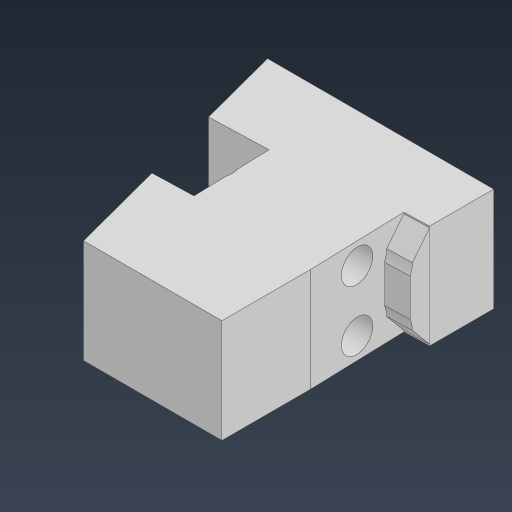
# Autodesk Inventor part: lunas_hold
Saved by Autodesk Inventor 2023 (Build 270158000, 158)
## iProperties
Created: 2026-01-11
Part Number: lunas_hold
Material: Generic
Document SubType Name: Modeling
Designer: szymo
Density: 1 g/cm^3
Appearance: Default
Author: szymo
Autodesk Inventor part; units mm, degrees
ref_plane "YZ Plane" through (0, 0, 0) normal (1, 0, 0) x (0, 1, 0)
ref_plane "XZ Plane" through (0, 0, 0) normal (0, 1, 0) x (-1, 0, 0)
ref_plane "XY Plane" through (0, 0, 0) normal (0, 0, 1) x (1, 0, 0)
ref_plane "Work Plane3" through (-37.2395, -29.2125, 19.3676) normal (0, -1, 0) x (0.9995066, 0, -0.0314108)
sketch "Sketch1" plane through (-37.2395, -29.2125, 19.3676) normal (0, -1, 0) x (0.9995066, 0, -0.0314108)
  line L0 (12, -4) -> (1, -4) construction
  line L1 (1, -4) -> (1, -14) construction
  line L2 (1, -14) -> (12, -14) construction
  line L3 (12, -14) -> (12, -13.8653) construction
  line L4 (10, -13.8653) -> (12, -13.8653) construction
  line L5 (10, -6.1347) -> (10, -13.8653) construction
  line L6 (10, -6.1347) -> (12, -6.1347) construction
  line L7 (12, -6.1347) -> (12, -4) construction
  line L8 (-5.9357, -19.5637) -> (1.1024, 11.0154) projected
  line L9 (1.1024, 11.0154) -> (32.2008, 11.9927) projected
  line L10 (33.1539, -18.3352) -> (32.2008, 11.9927) projected
  line L11 (33.1539, -18.3352) -> (-5.9357, -19.5637) projected
  line L12 (12.1612, -18.9949) -> (12, -13.8653)
  line L13 (12, -13.8653) -> (10, -13.8653)
  line L14 (10, -13.8653) -> (10, -6.1347)
  line L15 (10, -6.1347) -> (9.7777, 0.94)
  line L16 (-1.3163, -3.952) -> (-2.2908, -3.7277)
  line L17 (9.7777, 0.94) -> (-1.2966, 0.592)
  point P0 (37.8294, -18.1883)
  dimension "d0" = 20
  constraints: 12 end point, 2 perpendicular, 2 point on line, 1 collinear, 1 parallel, 3 other
  measures "d0" distance between parallel lines of L11 L17
extrude "Extrusion1" add sketch "Sketch1" along normal blind 8.3 contours L8 L17 L15 L14 L13 L12 L11
sketch "Sketch2" plane through (-27.4371, -37.5125, 12.9217) normal (0.9995066, 0, -0.0314108) x (-0.0314108, 0, -0.9995066)
  line L0 (7.7305, 8.3) -> (0, 8.3) projected
  line L1 (0, 8.3) -> (0, 0) projected
  line L2 (7.7305, 0) -> (0, 0) projected
  line L3 (7.7305, 8.3) -> (7.7305, 0) projected
  line L4 (-7.2847, -18.775) -> (-8.2847, -18.775) projected
  line L5 (-8.2847, -22.025) -> (-8.2847, -18.775) projected
  arc A0 (-8.2847, -22.025) -> (-7.7847, -22.525) centre (-7.7847, -22.025) ccw projected
  line L6 (-7.7847, -22.525) -> (-6.6313, -22.525) projected
  arc A1 (-6.1317, -23.0056) -> (-6.6313, -22.525) centre (-6.6313, -23.025) ccw projected
  arc A2 (-6.1317, -23.0056) -> (-2.1347, -26.85) centre (-2.1347, -22.85) ccw projected
  line L7 (0, -26.85) -> (-2.1347, -26.85) projected
  line L8 (1.6153, -28.775) -> (0, -26.85) projected
  arc A3 (1.6153, -28.775) -> (6.1153, -28.775) centre (3.8653, -28.775) ccw projected
  line L9 (7.7305, -26.85) -> (6.1153, -28.775) projected
  line L10 (7.8653, -26.85) -> (7.7305, -26.85) projected
  arc A4 (7.8653, -26.85) -> (12.8653, -21.85) centre (7.8653, -21.85) ccw projected
  line L11 (12.8653, -5.2) -> (12.8653, -21.85) projected
  arc A5 (12.8653, -5.2) -> (7.8653, -0.2) centre (7.8653, -5.2) ccw projected
  line L12 (7.7305, -0.2) -> (7.8653, -0.2) projected
  line L13 (6.1153, 1.725) -> (7.7305, -0.2) projected
  arc A6 (6.1153, 1.725) -> (1.6153, 1.725) centre (3.8653, 1.725) ccw projected
  line L14 (0, -0.2) -> (1.6153, 1.725) projected
  line L15 (-2.1347, -0.2) -> (0, -0.2) projected
  arc A7 (-2.1347, -0.2) -> (-6.1317, -4.0444) centre (-2.1347, -4.2) ccw projected
  arc A8 (-6.6313, -4.525) -> (-6.1317, -4.0444) centre (-6.6313, -4.025) ccw projected
  line L16 (-7.7847, -4.525) -> (-6.6313, -4.525) projected
  arc A9 (-7.7847, -4.525) -> (-8.2847, -5.025) centre (-7.7847, -5.025) ccw projected
  line L17 (-8.2847, -8.275) -> (-8.2847, -5.025) projected
  line L18 (-7.2847, -8.275) -> (-8.2847, -8.275) projected
  line L19 (-7.2847, -18.775) -> (-7.2847, -8.275) projected
  circle A10 centre (3.8653, -28.775) radius 1.1 projected
  circle A11 centre (3.8653, 1.725) radius 1.1 projected
  line L20 (-7.2847, 16.575) -> (-8.2847, 16.575) projected
  line L21 (-8.2847, 13.325) -> (-8.2847, 16.575) projected
  arc A12 (-8.2847, 13.325) -> (-7.7847, 12.825) centre (-7.7847, 13.325) ccw projected
  line L22 (-7.7847, 12.825) -> (-6.6313, 12.825) projected
  arc A13 (-6.1317, 12.3444) -> (-6.6313, 12.825) centre (-6.6313, 12.325) ccw projected
  arc A14 (-6.1317, 12.3444) -> (-2.1347, 8.5) centre (-2.1347, 12.5) ccw projected
  line L23 (0, 8.5) -> (-2.1347, 8.5) projected
  line L24 (1.6153, 6.575) -> (0, 8.5) projected
  arc A15 (1.6153, 6.575) -> (6.1153, 6.575) centre (3.8653, 6.575) ccw projected
  line L25 (7.7305, 8.5) -> (6.1153, 6.575) projected
  line L26 (7.8653, 8.5) -> (7.7305, 8.5) projected
  arc A16 (7.8653, 8.5) -> (12.8653, 13.5) centre (7.8653, 13.5) ccw projected
  line L27 (12.8653, 30.15) -> (12.8653, 13.5) projected
  arc A17 (12.8653, 30.15) -> (7.8653, 35.15) centre (7.8653, 30.15) ccw projected
  line L28 (7.7305, 35.15) -> (7.8653, 35.15) projected
  line L29 (6.1153, 37.075) -> (7.7305, 35.15) projected
  arc A18 (6.1153, 37.075) -> (1.6153, 37.075) centre (3.8653, 37.075) ccw projected
  line L30 (0, 35.15) -> (1.6153, 37.075) projected
  line L31 (-2.1347, 35.15) -> (0, 35.15) projected
  arc A19 (-2.1347, 35.15) -> (-6.1317, 31.3056) centre (-2.1347, 31.15) ccw projected
  arc A20 (-6.6313, 30.825) -> (-6.1317, 31.3056) centre (-6.6313, 31.325) ccw projected
  line L32 (-7.7847, 30.825) -> (-6.6313, 30.825) projected
  arc A21 (-7.7847, 30.825) -> (-8.2847, 30.325) centre (-7.7847, 30.325) ccw projected
  line L33 (-8.2847, 27.075) -> (-8.2847, 30.325) projected
  line L34 (-7.2847, 27.075) -> (-8.2847, 27.075) projected
  line L35 (-7.2847, 16.575) -> (-7.2847, 27.075) projected
  circle A22 centre (3.8653, 6.575) radius 1.1 projected
  circle A23 centre (3.8653, 37.075) radius 1.1 projected
  arc A24 (6.3141, 1.7991) -> (1.4164, 1.7991) centre (3.8653, 1.725) ccw
  line L36 (6.3141, 1.7991) -> (7.8238, 0)
  line L37 (7.8238, 0) -> (7.8653, 0)
  arc A25 (13.0653, -5.2) -> (7.8653, 0) centre (7.8653, -5.2) ccw
  line L38 (13.0653, -5.2) -> (13.0653, -21.85)
  arc A26 (7.8653, -27.05) -> (13.0653, -21.85) centre (7.8653, -21.85) ccw
  line L39 (7.8653, -27.05) -> (7.8238, -27.05)
  line L40 (7.8238, -27.05) -> (6.3141, -28.8491)
  arc A27 (1.4164, -28.8491) -> (6.3141, -28.8491) centre (3.8653, -28.775) ccw
  line L41 (1.4164, -28.8491) -> (-0.0933, -27.05)
  line L42 (-0.0933, -27.05) -> (-2.1347, -27.05)
  arc A28 (-6.3316, -23.0133) -> (-2.1347, -27.05) centre (-2.1347, -22.85) ccw
  arc A29 (-6.3316, -23.0133) -> (-6.6313, -22.725) centre (-6.6313, -23.025) ccw
  line L43 (-6.6313, -22.725) -> (-7.7847, -22.725)
  arc A30 (-8.4847, -22.025) -> (-7.7847, -22.725) centre (-7.7847, -22.025) ccw
  line L44 (-8.4847, -22.025) -> (-8.4847, -18.575)
  line L45 (-8.4847, -18.575) -> (-7.4847, -18.575)
  line L46 (-7.4847, -18.575) -> (-7.4847, -8.475)
  line L47 (-7.4847, -8.475) -> (-8.4847, -8.475)
  line L48 (-8.4847, -8.475) -> (-8.4847, -5.025)
  arc A31 (-7.7847, -4.325) -> (-8.4847, -5.025) centre (-7.7847, -5.025) ccw
  line L49 (-7.7847, -4.325) -> (-6.6313, -4.325)
  arc A32 (-6.6313, -4.325) -> (-6.3316, -4.0367) centre (-6.6313, -4.025) ccw
  arc A33 (-2.1347, 0) -> (-6.3316, -4.0367) centre (-2.1347, -4.2) ccw
  line L50 (-2.1347, 0) -> (-0.0933, 0)
  line L51 (-0.0933, 0) -> (1.4164, 1.7991)
  arc A34 (1.4164, 6.5009) -> (6.3141, 6.5009) centre (3.8653, 6.575) ccw
  line L52 (1.4164, 6.5009) -> (-0.0933, 8.3)
  line L53 (-0.0933, 8.3) -> (-2.1347, 8.3)
  arc A35 (-6.3316, 12.3367) -> (-2.1347, 8.3) centre (-2.1347, 12.5) ccw
  arc A36 (-6.3316, 12.3367) -> (-6.6313, 12.625) centre (-6.6313, 12.325) ccw
  line L54 (-6.6313, 12.625) -> (-7.7847, 12.625)
  arc A37 (-8.4847, 13.325) -> (-7.7847, 12.625) centre (-7.7847, 13.325) ccw
  line L55 (-8.4847, 13.325) -> (-8.4847, 16.775)
  line L56 (-8.4847, 16.775) -> (-7.4847, 16.775)
  line L57 (-7.4847, 16.775) -> (-7.4847, 26.875)
  line L58 (-7.4847, 26.875) -> (-8.4847, 26.875)
  line L59 (-8.4847, 26.875) -> (-8.4847, 30.325)
  arc A38 (-7.7847, 31.025) -> (-8.4847, 30.325) centre (-7.7847, 30.325) ccw
  line L60 (-7.7847, 31.025) -> (-6.6313, 31.025)
  arc A39 (-6.6313, 31.025) -> (-6.3316, 31.3133) centre (-6.6313, 31.325) ccw
  arc A40 (-2.1347, 35.35) -> (-6.3316, 31.3133) centre (-2.1347, 31.15) ccw
  line L61 (-2.1347, 35.35) -> (-0.0933, 35.35)
  line L62 (-0.0933, 35.35) -> (1.4164, 37.1491)
  arc A41 (6.3141, 37.1491) -> (1.4164, 37.1491) centre (3.8653, 37.075) ccw
  line L63 (6.3141, 37.1491) -> (7.8238, 35.35)
  line L64 (7.8238, 35.35) -> (7.8653, 35.35)
  arc A42 (13.0653, 30.15) -> (7.8653, 35.35) centre (7.8653, 30.15) ccw
  line L65 (13.0653, 30.15) -> (13.0653, 13.5)
  arc A43 (7.8653, 8.3) -> (13.0653, 13.5) centre (7.8653, 13.5) ccw
  line L66 (7.8653, 8.3) -> (7.8238, 8.3)
  line L67 (7.8238, 8.3) -> (6.3141, 6.5009)
  line L68 (6.1339, 2.65) -> (6.1339, 5.65)
  point P0 (12.0535, 37.5125)
  point P1 (7.7305, 0.1111)
  point P2 (7.7305, 8.1889)
  dimension "d3" = 0.2
  dimension "d4" = 0.2
  dimension "d5" = 3
  constraints: 66 end point, 42 point on circle, 20 centre point, 1 vertical, 50 other
  measures "d3" radial gap between concentric circles of A6 A24
  measures "d4" radial gap between concentric circles of A15 A34
  measures "d5" distance of L68.start L68.end
ref_plane "Work Plane4" through (-25.8422, -68.5375, 0) normal (0.9995066, 0, -0.0314108) x (0, 1, 0)
extrude "Extrusion2" add sketch "Sketch2" along normal up to surface (2 mm away) contours L3 L36 A24 L68 A34 L67
ref_plane "Work Plane5" through (-44.7843, -15.6875, 10.1) normal (0.9995066, 0, -0.0314108) x (0, 1, 0)
sketch "Sketch3" plane through (-44.7843, -15.6875, 10.1) normal (0.9995066, 0, -0.0314108) x (0, 1, 0)
  circle A0 centre (-20.1, -0.5) radius 1.1 projected
  circle A1 centre (-15.25, -0.5) radius 1.1 projected
  line L0 (-13.525, 10.092) -> (-13.525, -10.0637) projected
  line L1 (-13.525, 10.092) -> (-13.525, -10.0637) projected
  line L2 (-13.525, -10.0637) -> (-21.825, -10.0637) projected
  line L3 (-21.825, 10.092) -> (-21.825, -10.0637) projected
  line L4 (-13.525, 10.092) -> (-21.825, 10.092) projected
  line L5 (-21.825, -4.3653) -> (-21.825, 3.3653) projected
  line L6 (-13.525, 2.6) -> (-21.825, 2.6)
  line L7 (-21.825, 2.6) -> (-21.825, -3.6)
  line L8 (-21.825, -3.6) -> (-13.525, -3.6)
  line L9 (-13.525, -3.6) -> (-13.525, 2.6)
  point P0 (15.6875, -8.6883)
  point P1 (-21.825, -3.6)
  point P2 (-13.525, -3.6)
  point P3 (-13.525, 2.6)
  point P4 (-21.825, 2.6)
  dimension "d8" = 2
  dimension "d9" = 2
  constraints: 8 end point, 2 parallel, 2 point on line, 1 horizontal, 1 perpendicular
  measures "d8" distance edge to line of A1 L6
  measures "d9" distance edge to line of A1 L8
extrude "Extrusion3" cut sketch "Sketch3" along normal blind 7.5 contours A0 | A1 | L0 L8 L3 L6
sketch "Sketch4" plane through (-37.288, -15.6875, 9.8644) normal (-0.9995066, 0, 0.0314108) x (0.0314108, 0, 0.9995066)
  circle A0 centre (-0.5, -15.25) radius 1.1 projected
  circle A1 centre (-0.5, -20.1) radius 1.1 projected
  point P0 (-8.6883, 15.6875)
hole "Hole1" at (-37.3037, -30.9375, 9.3646) at (-37.3037, -35.7875, 9.3646) direction (0.9995066, 0, -0.0314108) diameter 2.6 end through all clearance for "Countersunk Flat Head Screw ISO 2009/7046" size "M2" standard "ISO"
chamfer "Chamfer1" distance 0.5 angle 45 2 edges at (-37.3425, -30.9375, 8.0652) (-37.3425, -35.7875, 8.0652)
sketch "Sketch5" plane through (-38.5169, -37.5125, 20) normal (-0.9669949, 0, 0.2547957) x (0.2547957, 0, 0.9669949)
  circle A0 centre (-7.1826, 49.9) radius 2.75 projected
  circle A1 centre (5.1959, 49.9) radius 2.75 projected
  line L0 (-14.05, 40.175) -> (-7.2389, 40.175) projected
  line L1 (-7.2389, 46.15) -> (-7.2389, 40.175) projected
  line L2 (10.6959, 46.15) -> (-7.2389, 46.15) projected
  line L3 (10.6959, 53.65) -> (10.6959, 46.15) projected
  line L4 (-20.6826, 53.65) -> (10.6959, 53.65) projected
  line L5 (-20.6826, 53.65) -> (-20.6826, 50.025) projected
  line L6 (-20.6826, 50.025) -> (-19.907, 50.025) projected
  line L7 (-19.907, 50.025) -> (-19.907, 35.35) projected
  line L8 (-14.05, 35.35) -> (-19.907, 35.35) projected
  line L9 (-14.05, 35.35) -> (-14.05, 40.175) projected
  line L10 (-7.6879, 8.3) -> (-7.6879, 0) projected
  line L11 (0, 0) -> (-7.6879, 0) projected
  line L12 (0, 8.3) -> (0, 0) projected
  line L13 (0, 8.3) -> (-7.6879, 8.3) projected
  circle A2 centre (-3.5, 4.15) radius 3.5
  point P0 (-9.526, 37.5125)
  dimension "d22" = 7
  dimension "d23" = 0.65
  dimension "d24" = 0.65
  dimension "d25" = 3.5
  constraints: 1 centre point
  measures "d22" diameter of A2
  measures "d23" distance edge to line of A2 L13
  measures "d24" distance edge to line of A2 L11
  measures "d25" distance from line of A2.centre L12
hole "Hole2" at (-39.4086, -33.3625, 16.6155) direction (0.9669949, 0, -0.2547957) diameter 4 depth 6 counterbore diameter 4.5 counterbore depth 1
sketch "Sketch6" plane through (-25.6809, -29.2125, 0) normal (0, 0, -1) x (-1, 0, 0)
  line L0 (18.1058, 0) -> (0, 0) projected
  line L1 (18.1058, -8.3) -> (0, -8.3) projected
  line L2 (18.1058, -33.825) -> (18.1058, 25.525) projected
  line L3 (0, 0) -> (0, -8.3) projected
  line L4 (1.7562, -8.3) -> (12.836, -8.3) projected
  line L5 (9.0529, -8.3) -> (9.0529, 0)
  line L6 (1.7562, 0) -> (12.836, 0) projected
  line L7 (18.1058, -8.3) -> (9.0529, 0)
  line L8 (0, -8.3) -> (9.0529, 0)
  line L9 (0, 0) -> (9.0529, -8.3)
  line L10 (18.1058, 0) -> (9.0529, -8.3)
  point P0 (-25.6809, 29.2125)
  point P1 (13.5793, -4.15)
  point P2 (4.5264, -4.15)
  dimension "d33" = 9.0529
  dimension "d34" = 9.0529
  constraints: 10 end point, 2 midpoint, 2 parallel, 2 point on line, 1 perpendicular
  measures "d33" distance between parallel lines of L2 L5
  measures "d34" distance between parallel lines of L5 L3
hole "Hole3" at (-39.2602, -33.3625, 0) at (-30.2073, -33.3625, 0) direction (0, 0, 1) diameter 4 depth 6 counterbore diameter 4.5 counterbore depth 1
equation "\"d23\" = d24"
equation "\"d25\" = 0.5 * d22"
equation "\"d33\" = d34"
body "Solid1"
